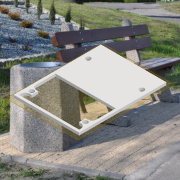
# Autodesk Inventor part: plytka
Saved by Autodesk Inventor 2021 (Build 250183000, 183)
## iProperties
Created: 2025-11-30
Part Number: plytka
Material: Generic
Document SubType Name: Modeling
Designer: huber
Density: 1 g/cm^3
Appearance: Default
Author: huber
Autodesk Inventor part; units mm, degrees
ref_plane "YZ Plane" through (0, 0, 0) normal (1, 0, 0) x (0, 1, 0)
ref_plane "XZ Plane" through (0, 0, 0) normal (0, 1, 0) x (-1, 0, 0)
ref_plane "XY Plane" through (0, 0, 0) normal (0, 0, 1) x (1, 0, 0)
ref_plane "Work Plane1" through (37.5, 25, 0) normal (0, 1, 0) x (-1, 0, 0)
sketch "Sketch1" plane through (37.5, 25, 0) normal (0, 1, 0) x (-1, 0, 0)
  line L0 (0, 0) -> (75, 0) projected
  line L1 (75, 0) -> (75, 100) projected
  line L2 (0, 100) -> (75, 100) projected
  line L3 (0, 0) -> (0, 100) projected
  circle A0 centre (6.75, 86) radius 2.7 projected
  circle A1 centre (68.25, 86) radius 2.7 projected
  circle A2 centre (68.25, 21.25) radius 2.7 projected
  circle A3 centre (6.75, 21.25) radius 2.7 projected
  line L4 (3, 3) -> (3, 17.5) projected
  line L5 (3, 17.5) -> (10.5, 17.5) projected
  line L6 (10.5, 17.5) -> (10.5, 25) projected
  line L7 (10.5, 25) -> (3, 25) projected
  line L8 (3, 25) -> (3, 77.25) projected
  arc A4 (8, 82.25) -> (3, 77.25) centre (8, 77.25) ccw projected
  line L9 (8, 82.25) -> (10.5, 82.25) projected
  line L10 (10.5, 82.25) -> (10.5, 89.75) projected
  line L11 (10.5, 89.75) -> (8, 89.75) projected
  arc A5 (3, 94.75) -> (8, 89.75) centre (8, 94.75) ccw projected
  line L12 (3, 94.75) -> (3, 97) projected
  line L13 (3, 97) -> (72, 97) projected
  line L14 (72, 97) -> (72, 94.75) projected
  arc A6 (67, 89.75) -> (72, 94.75) centre (67, 94.75) ccw projected
  line L15 (67, 89.75) -> (64.5, 89.75) projected
  line L16 (64.5, 89.75) -> (64.5, 82.25) projected
  line L17 (64.5, 82.25) -> (67, 82.25) projected
  arc A7 (72, 77.25) -> (67, 82.25) centre (67, 77.25) ccw projected
  line L18 (72, 77.25) -> (72, 25) projected
  line L19 (72, 25) -> (64.5, 25) projected
  line L20 (64.5, 25) -> (64.5, 17.5) projected
  line L21 (64.5, 17.5) -> (72, 17.5) projected
  line L22 (72, 17.5) -> (72, 3) projected
  line L23 (72, 3) -> (3, 3) projected
  line L24 (72, 55) -> (3, 55)
  point P0 (37.5, 0)
  dimension "d0" = 42
  constraints: 2 end point, 2 point on line, 1 perpendicular
  measures "d0" distance between parallel lines of L13 L24
extrude "Extrusion1" add sketch "Sketch1" along normal blind 3 contours L3 L2 L1 L0 | L4 L5 L6 L7 L8 L24 L18 L19 L20 L21 L22 L23
body "Solid1"
